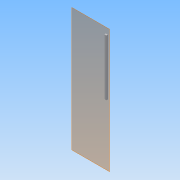
# Autodesk Inventor part: Sideborder
Saved by Autodesk Inventor 2013 (Build 170138000, 138)
## iProperties
Created: 2018-07-18
Part Number: Sideborder
Material: Generic
Document SubType Name: Modeling
Designer: Jeff Vyduna
Density: 1 g/cm^3
Author: Jeff Vyduna
Autodesk Inventor part; units mm, degrees
ref_plane "YZ Plane" through (0, 0, 0) normal (1, 0, 0) x (0, 1, 0)
ref_plane "XZ Plane" through (0, 0, 0) normal (0, 1, 0) x (-1, 0, 0)
ref_plane "XY Plane" through (0, 0, 0) normal (0, 0, 1) x (1, 0, 0)
ref_plane "Work Plane1" through (0, 0, 0) normal (0, 0, 1) x (1, 0, 0)
sketch "Sketch1" plane through (0, 0, 0) normal (0, 0, 1) x (1, 0, 0)
  line L0 (302.4187, 990.6) -> (264.3187, 990.6)
  line L1 (264.3187, 990.6) -> (264.3188, 0)
  line L2 (264.3188, 0) -> (302.4188, 0)
  line L3 (302.4188, 0) -> (302.4187, 990.6)
  point P0 (0, 0)
  dimension "d0" = 990.6
  dimension "d2" = 38.1
  constraints: 8 end point, 2 parallel, 1 coincident, 1 horizontal, 1 perpendicular, 1 other
  measures "d0" distance of L2.end L0.start
  measures "d2" distance of L0.start L0.end
extrude "Extrusion1" add sketch "Sketch1" along normal blind 25.4
sketch "Sketch2" plane through (0, 0, 25.4) normal (0, 0, 1) x (1, 0, 0)
  line L0 (264.3188, 0) -> (277.0187, 0)
  line L1 (277.0187, 0) -> (277.0187, 977.9)
  line L2 (277.0187, 977.9) -> (264.3187, 977.9)
  line L3 (264.3187, 977.9) -> (264.3188, 0)
  line L4 (302.4187, 990.6) -> (264.3187, 990.6) projected
  line L5 (264.3187, 990.6) -> (264.3188, 0) projected
  line L6 (264.3188, 0) -> (302.4188, 0) projected
  line L7 (302.4188, 0) -> (302.4187, 990.6) projected
  point P0 (0, 0)
  dimension "d5" = 977.9
  dimension "d7" = 12.7
  constraints: 8 end point, 2 parallel, 1 horizontal, 1 perpendicular
  measures "d5" distance of L0.end L1.end
  measures "d7" distance of L1.end L2.end
extrude "Extrusion2" cut sketch "Sketch2" against normal blind 8.4646 contours L3 L2 L1 L0
equation "\"d0\" = 0.5 * signH"
equation "\"d2\" = borderW"
equation "\"d3\" = borderH"
equation "\"d5\" = 0.5 * signH - panelLap"
equation "\"d7\" = panelLap"
equation "\"d8\" = panelH + velcroH + panelHClear"
equation "\"signH\" = 1981.2"
equation "\"borderW\" = 38.1"
equation "\"borderH\" = 25.4"
equation "\"velcroH\" = 2.54"
equation "\"panelH\" = 5.1308"
equation "\"panelHClear\" = 0.79375"
equation "\"panelLap\" = 12.7"
body "Solid1"
